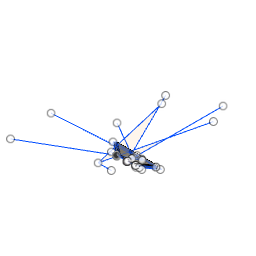
3Dplano v4 (Autodesk Fusion 360 design; units mm, degrees)
Autodesk Fusion 360 part; units mm, degrees
sketch "Sketch1" plane through (0, 0, 0) normal (0, 1, 0) x (1, 0, 0)
  line L0 (0, 0) -> (0, 239.8445)
  line L1 (0, 0) -> (0, 25)
  line L2 (0, 0) -> (-94.6434, 191.0764)
  line L3 (0, 0) -> (0, 15.4)
  line L4 (-10.6829, 21.5678) -> (-95.942, 70.7921)
  line L5 (13.3368, 23.1) -> (-199.4619, 9.5254)
  line L6 (-26.6736, 0) -> (-59.8805, 24.6504)
  line L7 (-33.0314, -39.3634) -> (-81.6324, 168.2553)
  line L8 (-33.0314, -39.3634) -> (21.6354, 194.1681)
  line L9 (-33.0314, -39.3634) -> (0, -39.3634)
  line L10 (-22.0861, 0.9535) -> (-23.3706, 1.907)
  line L11 (-49.9408, 21.6308) -> (-57.7944, 27.4607)
  line L12 (-23.3706, 1.907) -> (-46.756, 19.2666)
  line L13 (0, 15.4) -> (-10.6829, 21.5678)
  line L14 (-10.6829, 21.5678) -> (-14.9643, 24.0396)
  line L15 (0, 11.9359) -> (-12.1829, 18.9697)
  line L16 (-12.1829, 18.9697) -> (-16.4643, 21.4416)
  line L17 (-16.4643, 21.4416) -> (-14.9643, 24.0396)
  line L18 (-14.9643, 24.0396) -> (-59.0578, 24.0396)
  line L19 (-20.0907, 0.9577) -> (-19.0135, 2.4088)
  line L20 (-48.1526, 24.0396) -> (-49.9408, 21.6308)
  line L21 (-19.0135, 2.4088) -> (-21.5824, 4.3158)
  line L22 (-21.5824, 4.3158) -> (-44.9679, 21.6755)
  line L23 (-44.9679, 21.6755) -> (-48.1526, 24.0396)
  line L24 (-57.7944, 27.4607) -> (-56.0062, 29.8696)
  line L25 (-46.756, 19.2666) -> (-49.9408, 21.6308)
  line L26 (-48.1526, 24.0396) -> (-56.0062, 29.8696)
  line L27 (0, 0) -> (0, 1)
  line L28 (0, 1) -> (-20.0907, 0.9577)
  line L29 (13.3368, 23.1) -> (-20.5394, 3.5416)
  line L30 (-23.3706, 1.907) -> (-194.3746, -96.8223)
  line L31 (-20.5394, 3.5416) -> (-23.3706, 1.907)
  line L32 (-22.0861, 0.9535) -> (-20.298, 3.3623)
  line L33 (-20.0907, 0.9577) -> (-22.0861, 0.9535)
  line L34 (0, 0) -> (0, 25)
  line L35 (0, 1) -> (0, 2)
  line L36 (0, 2) -> (-19.317, 2)
  line L37 (-19.317, 2) -> (-19.3148, 0.9593)
  line L38 (46.756, 19.2666) -> (49.9408, 21.6308)
  line L39 (48.1526, 24.0396) -> (49.9408, 21.6308)
  line L40 (44.9679, 21.6755) -> (48.1526, 24.0396)
  line L41 (21.5824, 4.3158) -> (44.9679, 21.6755)
  line L42 (23.3706, 1.907) -> (46.756, 19.2666)
  line L43 (22.0861, 0.9535) -> (23.3706, 1.907)
  line L44 (20.0907, 0.9577) -> (19.0135, 2.4088)
  line L45 (19.0135, 2.4088) -> (21.5824, 4.3158)
  line L46 (20.0907, 0.9577) -> (22.0861, 0.9535)
  line L47 (0, 11.9359) -> (12.1829, 18.9697)
  line L48 (16.4643, 21.4416) -> (14.9643, 24.0396)
  line L49 (12.1829, 18.9697) -> (16.4643, 21.4416)
  line L50 (10.6829, 21.5678) -> (14.9643, 24.0396)
  line L51 (0, 15.4) -> (10.6829, 21.5678)
  line L52 (0, 1) -> (20.0907, 0.9577)
  line L53 (14.9643, 24.0396) -> (59.0578, 24.0396)
  line L54 (0, 2) -> (19.317, 2)
  line L55 (19.317, 2) -> (19.3148, 0.9593)
  line L56 (-14.9643, 24.0396) -> (14.9643, 24.0396)
  line L57 (0, 1) -> (35.9633, 0.9243)
  line L58 (0, 1) -> (-40.1034, 0.9577)
  line L59 (-23.8743, -1.4553) -> (-25.1587, -0.5018)
  line L60 (-25.1587, -0.5018) -> (-48.5442, 16.8578)
  line L61 (-48.5442, 16.8578) -> (-51.7289, 19.2219)
  line L62 (-51.7289, 19.2219) -> (-60.9132, 26.0396)
  line L63 (-14.9643, 26.0396) -> (-60.9132, 26.0396)
  line L64 (-14.9643, 26.0396) -> (14.9643, 26.0396)
  line L65 (14.9643, 26.0396) -> (60.9132, 26.0396)
  line L66 (23.8743, -1.4553) -> (25.1587, -0.5018)
  line L67 (25.1587, -0.5018) -> (48.5442, 16.8578)
  line L68 (28.529, 2) -> (60.9132, 26.0396)
  line L69 (18.4918, 0.9611) -> (18.4918, 2)
  line L70 (-18.5464, 0.9609) -> (-18.5464, 2)
  line L71 (19.1327, 2.2483) -> (21.7016, 4.1552)
  line L72 (21.7016, 4.1552) -> (45.0871, 21.5149)
  line L73 (45.0871, 21.5149) -> (48.2719, 23.879)
  line L74 (-0.1, 12.1091) -> (12.0829, 19.1429)
  line L75 (12.0829, 19.1429) -> (16.3643, 21.6148)
  line L76 (-0.05, 12.0225) -> (12.1329, 19.0563)
  line L77 (12.1329, 19.0563) -> (16.4143, 21.5282)
  line L78 (19.0731, 2.3285) -> (21.642, 4.2355)
  line L79 (21.642, 4.2355) -> (45.0275, 21.5952)
  line L80 (45.0275, 21.5952) -> (48.2123, 23.9593)
  dimension "d9" = 25
  dimension "d11" = 15.4
  dimension "d21" = 1
  dimension "d37" = 0.2
  dimension "d38" = 0.2
  dimension "d39" = 0.1
  dimension "d40" = 0.1
  measures "d11" distance of L0.start
  measures "d37" distance of L45
  measures "d38" distance of L47
  measures "d39" distance of L47
  measures "d40" distance of L45
extrude "Extrude2" add sketch "Sketch1" along normal blind 1 contours L0 L1 L3 L34 L35 L52 L54 L57 L69 | L0 L1 L3 L34 L40 L41 L44 L45 L47 L48 L49 L53 L54 | L52 L54 L55 L57 L69 | L0 L1 L3 L34 L47 L48 L49 L76 L77 | L44 L52 L55 L57 | L0 L1 L3 L34 L48 L74 L75 L76 L77 | L38 L39 L42 L43 L44 L46 L57 L71 L72 L73 | L0 L1 L3 L29 L34 L48 L50 L51 L74 L75 | L0 L1 L5 L29 L34 L50 L51 | L39 L44 L71 L72 L73 L78 L79 L80 | L38 L39 L42 L43 L53 L57 L67 L68 | L0 L1 L5 L34 L50 L56 | L39 L40 L41 L44 L45 L78 L79 L80 | L0 L1 L34 L53 L56 L64 L65 L68 makes body 1
extrude "Extrude3" add sketch "Sketch1" along normal blind 4 separate body contours L0 L1 L3 L34 L40 L41 L44 L45 L47 L48 L49 L53 L54 | L52 L54 L55 L57 L69 | L0 L1 L3 L34 L47 L48 L49 L76 L77 | L44 L52 L55 L57 | L0 L1 L5 L29 L34 L50 L51 | L38 L39 L42 L43 L53 L57 L67 L68 | L0 L1 L5 L34 L50 L56 | L39 L40 L41 L44 L45 L78 L79 L80 | L0 L1 L34 L53 L56 L64 L65 L68 makes body 2
mirror "Mirror1" about plane through (0, 0, 0) normal (1, 0, 0) of bodies 2 1 makes body 3 at (-27.6946, 4, -15.7863) makes body 4 at (-30.6791, 1, -14.9658)
combine "Combine1" operation add target body 4 tool bodies 3 2 1
fillet "Fillet2" radius 3.5 1 edges at (60.9132, 2, -26.0396) on bodies 4
fillet "Fillet3" radius 5.5 1 edges at (27.105, 2, -0.9429) on bodies 4
fillet "Fillet4" radius 5.5 1 edges at (-27.105, 2, -0.9429) on bodies 4
fillet "Fillet5" radius 3.5 1 edges at (-60.9132, 2, -26.0396) on bodies 4
equation "AA = 1.1 mm"
